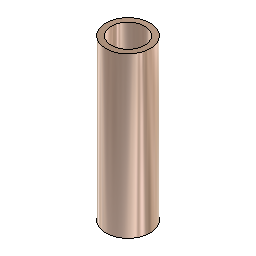
opjpcbprintheadassemblyv5 v15 (Autodesk Fusion 360 archive; units mm, degrees)
design "inletoutletpipes"
Autodesk Fusion 360 part; units mm, degrees
sketch "Sketch1" plane through (0, 0, 0) normal (0, 0, 1) x (1, 0, 0)
  circle A0 centre (0, 0) radius 2.5
  circle A1 centre (0, 0) radius 1.875
  dimension "d1" = 5
  dimension "d2" = 3.75
  constraint coincident A0.centre A1.centre
  constraint concentric A0 A1
  measures "d1" diameter of A0
  measures "d2" diameter of A1
extrude "Extrude1" add sketch "Sketch1" along normal blind 18

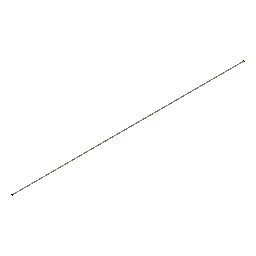
design "siliconcarbideheaterfilament"
Autodesk Fusion 360 part; units mm, degrees
sketch "Sketch1" plane through (0, 0, 0) normal (0, 1, 0) x (1, 0, 0)
  circle A0 centre (0, 0) radius 0.0675
  dimension "d1" = 0.135
  constraint coincident A0.centre origin
  measures "d1" diameter of A0
extrude "Extrude1" add sketch "Sketch1" along normal blind 37

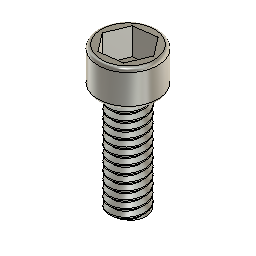
design "clampingfastenersstainlesssteelscrews"
Autodesk Fusion 360 part; units mm, degrees
sketch "Sketch1" plane through (0, 0, 0) normal (0, 0, 1) x (1, 0, 0)
  circle A0 centre (0, 0) radius 0.875
  dimension "d1" = 1.75
  constraint coincident A0.centre origin
  measures "d1" diameter of A0
extrude "Extrude1" add sketch "Sketch1" along normal blind 6.35
sketch "Sketch2" plane through (0, 0, 6.35) normal (0, 0, 1) x (-1, 0, 0)
  circle A0 centre (0, 0) radius 0.875
  circle A1 centre (0, 0) radius 1.775
  dimension "d4" = 3.55
  constraint coincident A0.centre A1.centre
  measures "d4" diameter of A1
extrude "Extrude2" add sketch "Sketch2" along normal blind 2.15 contours A0 | A1
thread "Thread1" "ANSI Unified Screw Threads 0.086(#2) 2-56 UNC 2A" major diameter 2.1184 minor diameter 1.6307 pitch 0.4536 angle 60 modelled right hand crest width 0.0713 on face at (0.8707, -0.0871, 4.2333) crest through (1.0592, 0, -0.1134)
sketch "Sketch3" plane through (0, 0, 8.5) normal (0, 0, 1) x (-1, 0, 0)
  circle A0 centre (0, 0) radius 1.775
  line L0 (-1.362, -0.1822) -> (-0.5232, -1.2706)
  line L1 (-0.5232, -1.2706) -> (0.8388, -1.0884)
  line L2 (0.8388, -1.0884) -> (1.362, 0.1822)
  line L3 (1.362, 0.1822) -> (0.5232, 1.2706)
  line L4 (0.5232, 1.2706) -> (-0.8388, 1.0884)
  line L5 (-0.8388, 1.0884) -> (-1.362, -0.1822)
  dimension "d7" = 1.19
  dimension "d8" = 1.362
  constraint coincident A0.centre origin
  measures "d7" distance of A0.centre L5
  measures "d8" horizontal distance of L0.end L1.end
extrude "Extrude3" cut sketch "Sketch3" against normal blind 1.6 contours L0 L1 L2 L3 L4 L5
fillet "Fillet1" radius 0.2 2 edges at (1.6549, 0.6419, 8.5) (1.6549, 0.6419, 6.35)

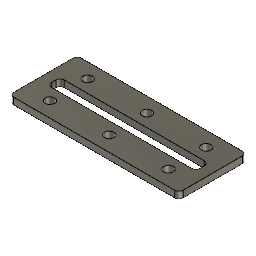
design "opjtankplatev5"
Autodesk Fusion 360 part; units mm, degrees
sketch "Sketch1" plane through (0, 0, 0) normal (0, 0, 1) x (1, 0, 0)
  line L0 (-20, 8) -> (20, 8)
  line L1 (20, 8) -> (20, -8)
  line L2 (20, -8) -> (-20, -8)
  line L3 (-20, -8) -> (-20, 8)
  line L4 (1.75, 0) -> (22.5, 0)
  line L5 (0, 1.75) -> (0, 22.5)
  dimension "d1" = 40
  dimension "d2" = 16
  constraint horizontal L0
  constraint vertical L1
  constraint horizontal L2
  constraint vertical L3
  constraint symmetric L0 L2 L4
  constraint symmetric L1 L3 L5
  measures "d1" distance of L0.start L0.end
  measures "d2" distance of L0.start L2.end
extrude "Extrude1" add sketch "Sketch1" along normal blind 1.6
sketch "Sketch2" plane through (0, 0, 1.6) normal (0, 0, 1) x (-1, 0, 0)
  line L0 (20, 8) -> (-20, 8)
  line L1 (-20, 8) -> (-20, -8)
  line L2 (-20, -8) -> (20, -8)
  line L3 (20, -8) -> (20, 8)
  line L4 (-1.75, 0) -> (-22.5, 0)
  line L5 (0, -1.75) -> (0, -22.5)
  circle A0 centre (0, -4.47) radius 1.115
  dimension "d5" = 2.23
  dimension "d6" = 3.53
  constraint coincident L5 A0.centre
  measures "d5" diameter of A0
  measures "d6" distance of L2 A0.centre
extrude "Extrude2" cut sketch "Sketch2" against normal through all contours L5 A0 | L5 A0
pattern_linear "R-Pattern1" count 3 spacing 13.97 along (1, 0, 0) both ways count 2 spacing 8.89 along (0, -1, 0) of "Extrude2"
sketch "Sketch3" plane through (0, 0, 1.6) normal (0, 0, 1) x (-1, 0, 0)
  circle A0 centre (-13.97, 4.42) radius 1.115
  circle A1 centre (0, 4.42) radius 1.115
  circle A2 centre (13.97, 4.42) radius 1.115
  circle A3 centre (-13.97, -4.47) radius 1.115
  circle A4 centre (13.97, -4.47) radius 1.115
  circle A5 centre (0, -4.47) radius 1.115
  line L0 (20, 8) -> (-20, 8)
  line L1 (-20, 8) -> (-20, -8)
  line L2 (-20, -8) -> (20, -8)
  line L3 (20, -8) -> (20, 8)
  line L4 (-17.5, 1.5) -> (17.5, 1.5)
  line L5 (17.5, 1.5) -> (17.5, -1.5)
  line L6 (17.5, -1.5) -> (-17.5, -1.5)
  line L7 (-17.5, -1.5) -> (-17.5, 1.5)
  line L8 (-17.5, 1.5) -> (17.5, -1.5) construction
  line L9 (17.5, 1.5) -> (-17.5, -1.5) construction
  dimension "d13" = 35
  dimension "d14" = 3
  constraint horizontal L4
  constraint perpendicular L4 L5
  constraint parallel L4 L6
  constraint parallel L5 L7
  constraint coincident L8 origin
  constraint coincident L9 origin
  measures "d13" distance of L5.end L6.end
  measures "d14" distance of L4.start L6.end
extrude "Extrude3" cut sketch "Sketch3" against normal through all contours L4 L5 L6 L7
fillet "Fillet1" radius 1 8 edges at (-20, -8, 0.8) (-20, 8, 0.8) (20, -8, 0.8) (20, 8, 0.8) (-17.5, 1.5, 0.8) (-17.5, -1.5, 0.8) (17.5, -1.5, 0.8) (17.5, 1.5, 0.8)
